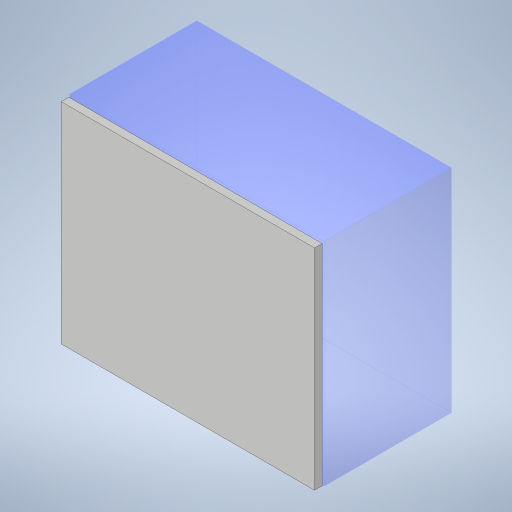
# Autodesk Inventor part: Horizontaly opening Door skeleton
Saved by Autodesk Inventor 2024 (Build 280153000, 153)
## iProperties
RuleStatus: InUse
Created: 2017-01-20
Part Number: Horizontaly opening Door skeleton
Material: Generic
Document SubType Name: Modeling
Designer: SvetlanaB
Density: 1 g/cm^3
Appearance: Default
Description: Horizontaly opening Door skeleton
Heigth: 500,000 mm
Width: 600,000 mm
Author: SvetlanaB
Autodesk Inventor part; units mm, degrees
ref_plane "YZ Plane" through (0, 0, 0) normal (1, 0, 0) x (0, 1, 0)
ref_plane "XZ Plane" through (0, 0, 0) normal (0, 1, 0) x (-1, 0, 0)
ref_plane "XY Plane" through (0, 0, 0) normal (0, 0, 1) x (1, 0, 0)
sketch "Sketch1" plane through (0, 0, 0) normal (0, 0, 1) x (1, 0, 0)
  line L0 (-300, 150) -> (300, 150)
  line L1 (300, 150) -> (300, -150)
  line L2 (300, -150) -> (-300, -150)
  line L3 (-300, -150) -> (-300, 150)
  line L4 (-300, 150) -> (300, -150) construction
  line L5 (300, 150) -> (-300, -150) construction
  point P0 (0, 0)
  dimension "Width" = 600
  dimension "Depth" = 300
  constraints: 12 end point, 2 midpoint, 2 parallel, 1 horizontal, 1 perpendicular
  measures "Width" distance of L1.end L2.end
  measures "Depth" distance between parallel lines of L2 L0
extrude "Extrusion1" add sketch "Sketch1" along normal blind 500
sketch "Sketch7" plane through (-300, -150, 0) normal (0, -1, 0) x (1, 0, 0)
  line L0 (600, 0) -> (0, 0) construction
  line L1 (600, 0) -> (600, 500) construction
  line L2 (0, 500) -> (600, 500) construction
  line L3 (0, 0) -> (0, 500) construction
  line L4 (1.5, 496) -> (598.5, 496)
  line L5 (598.5, 496) -> (598.5, 1.5)
  line L6 (598.5, 1.5) -> (1.5, 1.5)
  line L7 (1.5, 1.5) -> (1.5, 496)
  line L8 (600, 0) -> (0, 0)
  point P0 (300, 0)
  dimension "Offset_From_Top" = 4
  dimension "Offset_From_Right" = 1.5
  dimension "Offset_From_Left" = 1.5
  dimension "Offset_From_Bottom" = 1.5
  constraints: 10 end point, 2 parallel, 1 horizontal, 1 perpendicular
  measures "Offset_From_Top" distance between parallel lines of L4 L2
  measures "Offset_From_Right" distance between parallel lines of L1 L5
  measures "Offset_From_Left" distance between parallel lines of L3 L7
  measures "Offset_From_Bottom" distance between parallel lines of L0 L6
extrude "Extrusion7" add sketch "Sketch7" along normal blind 18 separate body
move or copy body "Move2" bodies to move or copy 2 copy no translate (0, -3, 0)
move or copy body "Move3" bodies to move or copy 2 copy no translate (0, 0.0001, 0)
equation "\"d37\" = Panel_thickness"
equation "\"Panel_thickness\" = 18"
